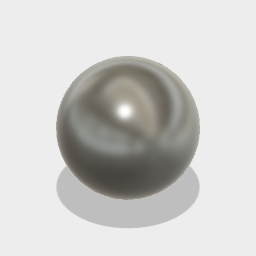
Ball (Autodesk Fusion 360 design; units mm, degrees)
Autodesk Fusion 360 part; units mm, degrees
sketch "Sketch1" plane through (0, 0, 0) normal (0, 1, 0) x (1, 0, 0)
  line L0 (0, 0) -> (0, -37)
  arc A0 (0, 37) -> (0, -37) centre (0, 0) ccw
  line L1 (0, 37) -> (0, 0)
  dimension "d2" = 37
  measures "d2" distance of L0.start L0.end
revolve "Revolve1" add sketch "Sketch1" angle 360 about axis through (0, 0, 0) along (0, 0, 1)
